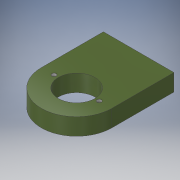
# Autodesk Inventor part: Bearing Housing
Saved by Autodesk Inventor 2018 (Build 220112000, 112)
## iProperties
Created: 2018-10-24
Part Number: Bearing Housing
Material: Generic
Document SubType Name: Modeling
Designer: iki
Density: 1 g/cm^3
Appearance: Default
Mass: 3.66114 g
Surface Area: 21.4665 cm^2
Volume: 3.66114 cm^3
Author: iki
Autodesk Inventor part; units mm, degrees
ref_plane "YZ Plane" through (0, 0, 0) normal (1, 0, 0) x (0, 1, 0)
ref_plane "XZ Plane" through (0, 0, 0) normal (0, 1, 0) x (-1, 0, 0)
ref_plane "XY Plane" through (0, 0, 0) normal (0, 0, 1) x (1, 0, 0)
sketch "Sketch1" plane through (0, 0, 0) normal (0, 0, 1) x (1, 0, 0)
  circle A0 centre (0, 0) radius 6.475
  arc A1 (-12.5, 0) -> (12.5, 0) centre (0, 0) ccw
  line L0 (-12.5, 0) -> (-12.5, 22)
  line L1 (-12.5, 22) -> (12.5, 22)
  line L2 (12.5, 22) -> (12.5, 0)
  dimension "d0" = 12.95
  dimension "d1" = 25
  dimension "d2" = 22
  dimension "d3" = 25
  constraints: 6 end point, 2 centre point, 2 coincident, 2 perpendicular, 2 point on circle, 1 tangent, 1 vertical
  measures "d0" diameter of A0
  measures "d1" diameter of A1
  measures "d2" distance of L0.start L0.end
  measures "d3" distance of L0.end L1.end
extrude "Extrusion1" add sketch "Sketch1" along normal blind 6
sketch "Sketch3" plane through (0, 0, 6) normal (0, 0, 1) x (1, 0, 0)
  circle A0 centre (-8, 0) radius 0.75
  circle A1 centre (8, 0) radius 0.75
  point P0 (0, 0)
  dimension "d7" = 16
  dimension "d8" = 8
  dimension "d9" = 1.5
  dimension "d10" = 1.5
  constraints: 2 centre point, 2 coincident
  measures "d7" distance of point (8, 0) point (-8, 0)
  measures "d8" distance of point (0, 0) point (-8, 0)
  measures "d9" diameter of A0
  measures "d10" diameter of A1
extrude "Extrusion2" cut sketch "Sketch3" against normal blind 8
body "Solid1"
